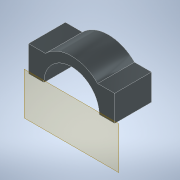
# Autodesk Inventor part: Крышка коренного подшипника1
Saved by Autodesk Inventor 2021 (Build 250183000, 183)
## iProperties
Created: 2020-12-05
Part Number: Крышка коренного подшипника1
Material: Чугун, серый
Document SubType Name: Modeling
Designer: Тимоха
Mass: 13008.4 g
Surface Area: 1324.92 cm^2
Volume: 1819.36 cm^3
Density: 7.15 g/cm^3
Appearance: Чугун серый
Author: Тимоха
Autodesk Inventor part; units mm, degrees
ref_plane "YZ Plane" through (0, 0, 0) normal (1, 0, 0) x (0, 1, 0)
ref_plane "XZ Plane" through (0, 0, 0) normal (0, 1, 0) x (-1, 0, 0)
ref_plane "XY Plane" through (0, 0, 0) normal (0, 0, 1) x (1, 0, 0)
ref_plane "РабПлоскость1" through (0, 0, 0) normal (0, 0, 1) x (1, 0, 0)
sketch "Эскиз1" plane through (0, 0, 0) normal (0, 0, 1) x (1, 0, 0)
  arc A0 (-90, 62.5) -> (90, 62.5) centre (0, 62.5) ccw projected
  circle A1 centre (0, 62.5) radius 90
  line L0 (-140, 62.5) -> (-90, 62.5) projected
  line L1 (90, 62.5) -> (140, 62.5) projected
  line L2 (-140, 62.5) -> (-140, 147.5)
  line L3 (-140, 147.5) -> (-29.5804, 147.5)
  line L4 (140, 62.5) -> (140, 147.5)
  line L5 (140, 147.5) -> (29.5804, 147.5)
  circle A2 centre (0, 62.5) radius 120
  point P0 (0, 0)
  point P1 (84.7054, 147.5)
  point P2 (-84.7054, 147.5)
  dimension "d0" = 85
  dimension "d1" = 240
  constraints: 8 end point, 2 centre point, 2 coincident, 2 perpendicular, 2 point on circle, 2 point on line, 1 vertical
  measures "d0" distance of L0.start L2.end
  measures "d1" diameter of A2
extrude "Выдавливание1" add sketch "Эскиз1" against normal blind 120 contours L0 A2 L3 A1 | A1 L5 A2 L1 | L3 A2 L5 A1 | L0 L2 L3 A2 | A2 L5 L4 L1
sketch "Эскиз2" plane through (84.7054, 147.5, 0) normal (0, 1, 0) x (1, 0, 0)
  line L0 (55.2946, 0) -> (0, 0) projected
  line L1 (55.2946, 0) -> (55.2946, 120) projected
  line L2 (0, 120) -> (55.2946, 120) projected
  line L3 (0, 0) -> (0, 120) projected
  circle A0 centre (27.6473, 60) radius 12.5
  point P0 (-84.7054, 0)
  dimension "d4" = 25
  constraints: 1 centre point
  measures "d4" diameter of A0
extrude "Выдавливание2" cut sketch "Эскиз2" against normal blind 85 contours A0
mirror "Зеркальное отражение1" about plane through (0, 0, 0) normal (1, 0, 0) of "Выдавливание2"
